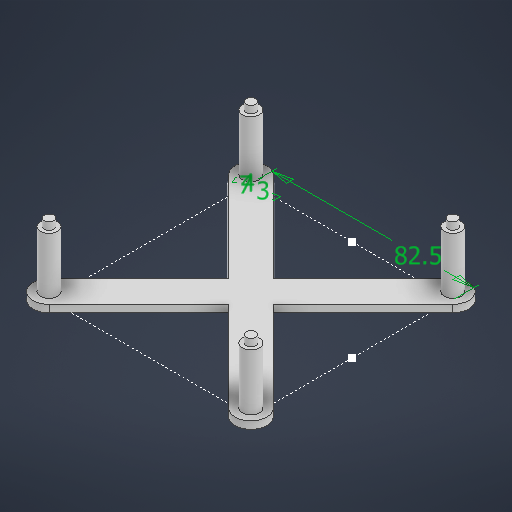
# Autodesk Inventor part: ConformalCoatingJig
Saved by Autodesk Inventor 2026 (Build 300175050, 175E)
## iProperties
Created: 2025-08-10
Part Number: ConformalCoatingJig
Material: Generic
Document SubType Name: Modeling
Designer: user
Density: 1 g/cm^3
Appearance: Default
Author: user
## iProperties of the stored document ConformalCoatingJig_3DPrint.ipt
Created: 2025-08-10
Part Number: ConformalCoatingJig_3DPrint
Material: Generic
Document SubType Name: Modeling
Designer: user
Density: 1 g/cm^3
Appearance: Default
Author: user
Autodesk Inventor part; units mm, degrees
ref_plane "YZ Plane" through (0, 0, 0) normal (1, 0, 0) x (0, 1, 0)
ref_plane "XZ Plane" through (0, 0, 0) normal (0, 1, 0) x (-1, 0, 0)
ref_plane "XY Plane" through (0, 0, 0) normal (0, 0, 1) x (1, 0, 0)
sketch "Sketch1" plane through (0, 0, 0) normal (0, 1, 0) x (-1, 0, 0)
  line L0 (41.25, -41.25) -> (-41.25, -41.25) construction
  line L1 (-41.25, -41.25) -> (-41.25, 41.25) construction
  line L2 (-41.25, 41.25) -> (41.25, 41.25) construction
  line L3 (41.25, 41.25) -> (41.25, -41.25) construction
  circle A0 centre (41.25, -41.25) radius 3.5
  circle A1 centre (41.25, -41.25) radius 2
  circle A2 centre (41.25, -41.25) radius 6.5
  line L4 (45.8462, -36.6538) -> (4.5962, 4.5962)
  line L5 (4.5962, 4.5962) -> (-4.5962, -4.5962)
  line L6 (-4.5962, -4.5962) -> (36.6538, -45.8462)
  point P0 (0, 0)
  point P1 (0, -41.25)
  point P2 (-41.25, 0)
  point P3 (0, 0)
  dimension "d0" = 82.5
  dimension "d1" = 4
  dimension "d2" = 7
  dimension "d3" = 3
  constraints: 14 end point, 3 centre point, 3 coincident, 3 midpoint, 3 parallel, 3 perpendicular, 2 point on circle, 2 tangent, 1 horizontal, 1 horizontal alignment, 1 vertical alignment
  measures "d0" distance of L0.start L0.end
  measures "d1" diameter of A1
  measures "d2" diameter of A0
  measures "d3" radial gap between concentric circles of A0 A2
extrude "Extrusion1" add sketch "Sketch1" along normal blind 3 contours A2 L6 L5 L4
extrude "Extrusion2" add sketch "Sketch1" along normal blind 29 contours A1
extrude "Extrusion3" add sketch "Sketch1" along normal blind 26 contours A0
extrude "Extrusion4" add sketch "Sketch1" along normal blind 3 contours A2
pattern_circular "Circular Pattern1" count 4 over 360 about axis through (0, -10, 0) along (0, 1, 0) of "Extrusion1", "Extrusion2", "Extrusion3", "Extrusion4"
body "Solid1"
